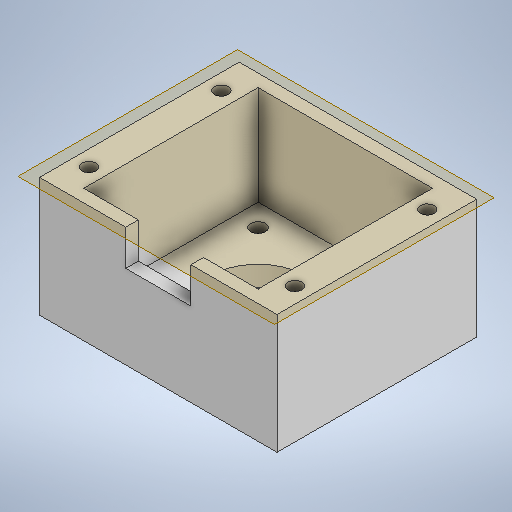
# Autodesk Inventor part: motor_case2
Saved by Autodesk Inventor 2025.1 (Build 291241000, 241)
## iProperties
Created: 2024-11-25
Part Number: motor_case2
Material: 一般
Document SubType Name: Modeling
Designer: dell
Density: 1 g/cm^3
Appearance: 既定
Author: dell
Autodesk Inventor part; units mm, degrees
ref_plane "YZ Plane" through (0, 0, 0) normal (1, 0, 0) x (0, 1, 0)
ref_plane "XZ Plane" through (0, 0, 0) normal (0, 1, 0) x (-1, 0, 0)
ref_plane "XY Plane" through (0, 0, 0) normal (0, 0, 1) x (1, 0, 0)
sketch "スケッチ1" plane through (0, 0, 0) normal (0, 1, 0) x (-1, 0, 0)
  line L0 (0, 0) -> (-56.5, 0)
  line L1 (-56.5, 0) -> (-56.5, -47.5)
  line L2 (-56.5, -47.5) -> (0, -47.5)
  line L3 (0, -47.5) -> (0, 0)
  line L4 (-7.5, -3) -> (-49, -3)
  line L5 (-49, -3) -> (-49, -44.5)
  line L6 (-49, -44.5) -> (-7.5, -44.5)
  line L7 (-7.5, -44.5) -> (-7.5, -3)
  dimension "d0" = 56.5
  dimension "d1" = 47.5
  dimension "d6" = 41.5
  dimension "d7" = 41.5
  constraints: 16 end point, 4 parallel, 2 horizontal, 2 perpendicular
  measures "d0" distance of L2.end L1.end
  measures "d1" distance of L1.end L0.end
  measures "d6" distance of L6.end L5.end
  measures "d7" distance of L5.end L4.end
extrude "押し出し1" add sketch "スケッチ1" along normal blind 28.4 contours L3 L2 L1 L0 | L7 L6 L5 L4
ref_plane "作業平面2" through (0, 28.4, 0) normal (0, 1, 0) x (1, 0, 0)
sketch "スケッチ3" plane through (0, 28.4, 0) normal (0, 1, 0) x (1, 0, 0)
  line L0 (7.5, 3) -> (49, 3)
  line L1 (49, 3) -> (49, 44.5)
  line L2 (49, 44.5) -> (7.5, 44.5)
  line L3 (7.5, 44.5) -> (7.5, 3)
  point P0 (0, 0)
  dimension "d8" = 41.5
  dimension "d9" = 41.5
  constraints: 8 end point, 2 parallel, 1 horizontal, 1 perpendicular
  measures "d8" distance of L2.end L1.end
  measures "d9" distance of L1.end L0.end
extrude "押し出し2" cut sketch "スケッチ3" against normal blind 23.6
sketch "スケッチ4" plane through (0, 4.8, 0) normal (0, 1, 0) x (1, 0, 0)
  line L0 (7.5, 3) -> (7.5, 44.5) projected
  line L1 (49, 44.5) -> (49, 3) projected
  line L2 (7.5, 44.5) -> (49, 44.5) projected
  point P0 (0, 0)
  point P1 (28.25, 23.75)
hole "穴1" at (28.25, 4.8, -23.75) direction (0, -1, 0) diameter 22.5 end through all
sketch "スケッチ5" plane through (0, 4.8, 0) normal (0, 1, 0) x (1, 0, 0)
  line L0 (7.5, 44.5) -> (49, 44.5) projected
  line L1 (7.5, 3) -> (7.5, 44.5) projected
  line L2 (49, 44.5) -> (49, 3) projected
  line L3 (49, 3) -> (7.5, 3) projected
  point P0 (0, 0)
  point P1 (12.75, 39.25)
  point P2 (43.75, 39.25)
  point P3 (43.75, 8.25)
  point P4 (12.75, 8.25)
  dimension "d23" = 5.25
  dimension "d24" = 5.25
  dimension "d25" = 5.25
  dimension "d26" = 5.25
  dimension "d27" = 5.25
  dimension "d28" = 5.25
  dimension "d29" = 5.25
  dimension "d30" = 5.25
  measures "d23" distance from line of L0 point (12.75, 39.25)
  measures "d24" distance from line of L1 point (12.75, 39.25)
  measures "d25" distance from line of L2 point (43.75, 39.25)
  measures "d26" distance from line of L0 point (43.75, 39.25)
  measures "d27" distance from line of L2 point (43.75, 8.25)
  measures "d28" distance from line of L3 point (43.75, 8.25)
  measures "d29" distance from line of L3 point (12.75, 8.25)
  measures "d30" distance from line of L1 point (12.75, 8.25)
hole "穴2" at (12.75, 4.8, -39.25) at (43.75, 4.8, -39.25) at (43.75, 4.8, -8.25) at (12.75, 4.8, -8.25) direction (0, -1, 0) diameter 3.5 end through all
sketch "スケッチ6" plane through (0, 28.4, 0) normal (0, 1, 0) x (1, 0, 0)
  line L0 (0, 47.5) -> (0, 0) projected
  line L1 (49, 44.5) -> (49, 3) projected
  line L2 (56.5, 47.5) -> (0, 47.5) projected
  line L3 (0, 0) -> (56.5, 0) projected
  line L4 (56.5, 0) -> (56.5, 47.5) projected
  point P0 (3.75, 39.5)
  point P1 (3.75, 8)
  point P2 (52.75, 8)
  point P3 (52.75, 39.5)
  dimension "d38" = 3.75
  dimension "d40" = 8
  dimension "d41" = 8
  dimension "d42" = 3.75
  dimension "d43" = 3.75
  dimension "d44" = 8
  dimension "d45" = 8
  dimension "d46" = 3.75
  measures "d38" distance from line of L0 point (3.75, 39.5)
  measures "d40" distance from line of L2 point (3.75, 39.5)
  measures "d41" distance from line of L3 point (3.75, 8)
  measures "d42" distance from line of L0 point (3.75, 8)
  measures "d43" distance from line of L4 point (52.75, 8)
  measures "d44" distance from line of L3 point (52.75, 8)
  measures "d45" distance from line of L2 point (52.75, 39.5)
  measures "d46" distance from line of L4 point (52.75, 39.5)
hole "穴3" at (3.75, 28.4, -39.5) at (3.75, 28.4, -8) at (52.75, 28.4, -8) at (52.75, 28.4, -39.5) direction (0, -1, 0) diameter 3.3 depth 15
sketch "スケッチ7" plane through (0, 0, 0) normal (0, 0, 1) x (1, 0, 0)
  line L0 (56.5, 28.4) -> (0, 28.4) projected
  line L1 (20.5, 28.4) -> (36, 28.4)
  line L2 (36, 28.4) -> (36, 19.9)
  line L3 (36, 19.9) -> (20.5, 19.9)
  line L4 (20.5, 19.9) -> (20.5, 28.4)
  line L5 (0, 0) -> (56.5, 0) projected
  dimension "d55" = 15.5
  constraints: 8 end point, 2 parallel, 1 horizontal, 1 perpendicular, 1 point on line
  measures "d55" distance of L2.end L3.end
extrude "押し出し3" cut sketch "スケッチ7" against normal blind 3
